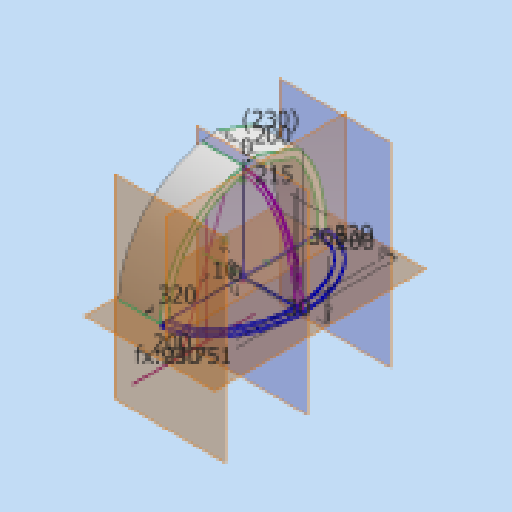
# Autodesk Inventor part: eggshell_3dprintcore
Saved by Autodesk Inventor 2023 (Build 270158000, 158)
## iProperties
Created: 2026-03-19
Part Number: eggshell_3dprintcore
Material: Generic
Document SubType Name: Modeling
Designer: Nathann
Density: 1 g/cm^3
Appearance: Default
Author: Nathann
Autodesk Inventor part; units mm, degrees
ref_plane "YZ Plane" through (0, 0, 0) normal (1, 0, 0) x (0, 1, 0)
ref_plane "XY Plane" through (0, 0, 0) normal (0, 0, 1) x (1, 0, 0)
sketch "Sketch2" plane through (0, 0, 0) normal (1, 0, 0) x (0, 1, 0)
  line L0 (0, 380) -> (0, 410)
  line L1 (0, -230) -> (0, -200)
  line L2 (0, 0) -> (0, 132.8644)
  line L3 (295.6158, -112.924) -> (350.339, 37.4268)
  line L4 (379.3536, 29.4296) -> (324.6304, -120.9212)
  ellipse E0 centre (0, 0) end of major axis (358.1699, 0) minor radius 200 (0, -200) -> (295.6158, -112.924) ccw
  ellipse E1 centre (0, 0) end of major axis (352.0508, 0) minor radius 380 (350.339, 37.4268) -> (0, 380) ccw
  ellipse E2 centre (0, 0) end of major axis (381.6296, 0) minor radius 230 (0, -230) -> (324.6304, -120.9212) ccw
  ellipse E3 centre (0, 0) end of major axis (380.3347, 0) minor radius 410 (379.3536, 29.4296) -> (0, 410) ccw
  point P0 (0, 0)
  dimension "d10" = 30
  dimension "d11" = 30
  dimension "d12" = 0
  dimension "d16" = 380
  dimension "d17" = 200
  dimension "d25" = 20
  dimension "d26" = 160
  dimension "d27" = 30
  dimension "d28" = 160
  constraints: 11 end point, 4 vertical, 2 coincident, 2 point on line, 1 parallel, 16 other
  measures "d10" distance of L0.start L0.end
  measures "d11" distance of L1.start L1.end
  measures "d12" distance from line of point (0, 0) L0
  measures "d16" distance of point (0, 0) L0.start
  measures "d17" distance of L1.end point (0, 0)
  measures "d25" angle of L2 L3
  measures "d26" distance of L3.start L3.end
  measures "d27" distance between parallel lines of L4 L3
  measures "d28" distance of L4.start L4.end
extrude "Extrusion1" add sketch "Sketch2" along normal blind 160
sketch "Sketch3" plane through (0, 0, 0) normal (-1, 0, 0) x (0, 0, 1)
  line L0 (171.5389, -307.9404) -> (-54.4979, 313.0907)
  line L1 (-120.9212, 324.6304) -> (29.4296, 379.3536) projected
  line L2 (-111.428, -307.9404) -> (360.7046, -307.9404)
  line L3 (76.7879, 236.8347) -> (76.7879, -307.9404)
  point P0 (0, 0)
  dimension "d31" = 94.751
  constraints: 6 end point, 2 perpendicular, 1 horizontal, 1 point on line
  measures "d31" distance of L0.start L3.end
sketch "Sketch4" plane through (0, 0, 380) normal (0, -1, 0) x (1, 0, 0)
  line L0 (160, 30) -> (160, 0) projected
  line L1 (160, -610) -> (160, -500.9212) projected
  line L2 (160, 30) -> (160, -610)
  line L3 (160, 0) -> (160, -342.5732) projected
  ellipse E0 centre (160, -290) end of major axis (390, -290) minor radius 320 (160, -610) -> (160, 30) ccw
  line L4 (0, 30) -> (160, 30) projected
  line L5 (0, 0) -> (160, 0) projected
  ellipse E1 centre (160, -290) end of major axis (360, -290) minor radius 290 (160, -580) -> (160, 0) ccw
  point P0 (0, -380)
  dimension "d33" = 200
  dimension "d34" = 230
  dimension "d32" = 320
  constraints: 4 end point, 3 point on line, 1 coincident, 1 collinear, 1 vertical, 8 other
  measures "d32" distance from line of L4 point (160, -290)
ref_plane "Work Plane3" through (0, 0, 90) normal (0, 0, -1) x (-1, 0, 0)
ref_plane "Work Plane1" through (0, 0, -230) normal (0, 0, -1) x (-1, 0, 0)
ref_plane "Work Plane2" through (0, 0, 410) normal (0, 0, 1) x (1, 0, 0)
sketch "Sketch6" plane through (0, 0, 90) normal (0, 0, -1) x (-1, 0, 0)
  line L0 (-160, 371.0583) -> (0, 371.0583) projected
  line L1 (0, 371.0583) -> (0, 342.0343) projected
  line L2 (0, 342.0343) -> (-160, 342.0343) projected
  line L3 (-160, 342.0343) -> (-160, 371.0583) projected
  ellipse E0 centre (-160, -10) end of major axis (-390, -10) minor radius 381.0583 (-160, 371.0583) -> (-390, -10) ccw
  line L4 (-160, 0) -> (-160, 350.339) projected
  line L5 (-160, 342.0343) -> (-160, 371.0583)
  line L6 (-360, -10) -> (-390, -10)
  ellipse E1 centre (-160, -10) end of major axis (-360, -10) minor radius 352.0343 (-160, 342.0343) -> (-360, -10) ccw
  ellipse E2 centre (-160, -10) end of major axis (-403.0676, -10) minor radius 410.7244 (-34.7861, 342.0343) -> (-69.2995, 371.0583) ccw
  line L7 (0, 0) -> (-160, 0) projected
  point P0 (-160, 324.6304)
  dimension "d62" = 200
  dimension "d63" = 230
  dimension "d58" = 30
  dimension "d59" = 0
  dimension "d60" = 10
  dimension "d61" = 0
  constraints: 4 end point, 3 point on line, 2 vertical, 1 coincident, 1 horizontal, 12 other
  measures "d58" distance of L6.start L6.end
  measures "d59" distance from line of point (-160, -10) L6
  measures "d60" distance from line of L7 point (-160, -10)
  measures "d61" distance from line of point (-160, -10) L5
sketch "Sketch7" plane through (0, 0, 90) normal (0, 0, -1) x (-1, 0, 0)
  line L0 (0, 0) -> (-160, 0) projected
  ellipse E0 centre (-160, 0) end of major axis (-160, 365) minor radius 215 (-160, 365) -> (-375, 0) ccw
  line L1 (-160, 0) -> (-160, 350.339) projected
  line L2 (-375, 0) -> (-160, 0)
  line L3 (-160, 0) -> (-160, 365)
  line L4 (-160, 324.6304) -> (-160, 379.3536) projected
  dimension "d40" = 215
  dimension "d41" = 365
  constraints: 4 end point, 1 horizontal, 1 point on line, 4 other
ref_plane "Work Plane4" through (210, 0, 0) normal (1, 0, 0) x (0, 0, -1)
sketch "Sketch10" plane through (160, 0, 0) normal (1, 0, 0) x (0, 0, -1)
  line L0 (120.9212, 324.6304) -> (-29.4296, 379.3536) projected
  ellipse E0 centre (0, 0) end of major axis (-410, 0) minor radius 380.3347 (-29.4296, 379.3536) -> (-410, 0) ccw projected
  line L1 (-410, 0) -> (-380, 0) projected
  ellipse E1 centre (0, 0) end of major axis (-380, 0) minor radius 352.0508 (-37.4268, 350.339) -> (-380, 0) ccw projected
  line L2 (-37.4268, 350.339) -> (112.924, 295.6158) projected
  ellipse E2 centre (0, 0) end of major axis (0, -358.1699) minor radius 200 (200, 0) -> (112.924, 295.6158) ccw projected
  line L3 (200, 0) -> (230, 0) projected
  ellipse E3 centre (0, 0) end of major axis (0, 381.6296) minor radius 230 (230, 0) -> (120.9212, 324.6304) ccw projected
  point P0 (0, 0)
  constraints: 4 other
ref_plane "Work Plane5" through (0, -10, 0) normal (0, 1, 0) x (-1, 0, 0)
sketch "Sketch11" plane through (0, -10, 0) normal (0, 1, 0) x (-1, 0, 0)
  line L0 (-160, -200) -> (-160, -230) projected
  ellipse E0 centre (-160, 90) end of major axis (-160, -230) minor radius 230 (-160, 410) -> (-160, -230) ccw
  line L1 (-160, -200) -> (-160, -112.924) projected
  ellipse E1 centre (-160, 90) end of major axis (-160, -200) minor radius 200 (-160, 380) -> (-160, -200) ccw
  line L2 (0, -230) -> (-160, -230) projected
  line L3 (-160, -200) -> (-160, -230)
  line L4 (0, 380) -> (-160, 380) projected
  line L5 (-160, 410) -> (-160, 380)
  line L6 (-160, 380) -> (-160, 410)
  point P0 (0, 0)
  dimension "d48" = 230
  dimension "d49" = 200
  constraints: 6 end point, 5 vertical, 2 coincident, 8 other
equation "\"d28\" = d26"
body "Solid1"
